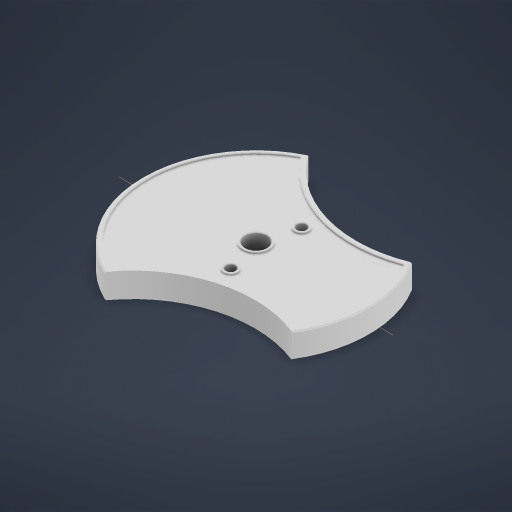
# Autodesk Inventor part: Disk
Saved by Autodesk Inventor 2023.2 (Build 272271000, 271)
## iProperties
Created: 2022-11-28
Part Number: Disk
Material: Generic
Document SubType Name: Modeling
Designer: iusti
Density: 1 g/cm^3
Appearance: Gunmetal - Antique Polished
Author: iusti
Autodesk Inventor part; units mm, degrees
ref_plane "YZ Plane" through (0, 0, 0) normal (1, 0, 0) x (0, 1, 0)
ref_plane "XZ Plane" through (0, 0, 0) normal (0, 1, 0) x (-1, 0, 0)
ref_plane "XY Plane" through (0, 0, 0) normal (0, 0, 1) x (1, 0, 0)
sketch "Sketch1" plane through (0, 0, 0) normal (0, 1, 0) x (-1, 0, 0)
  arc A0 (-38.9896, 24.4092) -> (-38.9896, -24.4092) centre (0, 0) ccw
  arc A1 (-38.9896, 24.4092) -> (20.1302, 41.3615) centre (-20.1215, 70.1721) ccw
  line L0 (0, 0) -> (-20.1215, 70.1721) construction
  line L1 (102.2, 0) -> (-102.2, 0) construction
  circle A2 centre (0, 0) radius 73 construction
  arc A3 (20.1302, -41.3615) -> (-38.9896, -24.4092) centre (-20.1215, -70.1721) ccw
  line L2 (20.1302, 41.3615) -> (20.1302, -41.3615) construction
  line L3 (-38.9896, 24.4092) -> (-38.9896, -24.4092) construction
  arc A4 (-12.6793, 44.218) -> (-38.9896, 24.4092) centre (0, 0) ccw construction
  arc A5 (20.1302, 41.3615) -> (-12.6793, 44.218) centre (0, 0) ccw construction
  arc A6 (20.1302, -41.3615) -> (20.1302, 41.3615) centre (0, 0) ccw
  arc A7 (-38.9896, -24.4092) -> (20.1302, -41.3615) centre (0, 0) ccw construction
  dimension "d3" = 146
  dimension "d0" = 92
  dimension "d1" = 49.5
  dimension "d2" = 74
  constraints: 14 point on circle, 7 centre point, 6 end point, 3 coincident, 3 symmetric about line, 2 vertical, 1 point on line, 4 other
  measures "d0" diameter of A0
  measures "d1" radius of A1
  measures "d2" angle of L1 L0
extrude "Extrusion1" add sketch "Sketch1" along normal mid plane 10
sketch "Sketch6" plane through (0, 5, 0) normal (0, 1, 0) x (1, 0, 0)
  arc A0 (-20.1302, 41.3615) -> (-20.1302, -41.3615) centre (0, 0) ccw projected
  arc A1 (38.9896, -24.4092) -> (-20.1302, -41.3615) centre (20.1215, -70.1721) ccw projected
  arc A2 (38.9896, -24.4092) -> (38.9896, 24.4092) centre (0, 0) ccw projected
  arc A3 (-20.1302, 41.3615) -> (38.9896, 24.4092) centre (20.1215, 70.1721) ccw projected
  line L0 (0, 0) -> (20.1215, -70.1721) construction
  line L1 (0, 0) -> (20.1215, 70.1721) construction
  point P0 (4.1346, -14.4189)
  point P1 (4.1346, 14.4189)
  dimension "d15" = 15
  constraints: 4 end point, 2 point on line, 1 vertical alignment
  measures "d15" distance of point (4.135, -14.419) A0.centre
hole "Hole1" at (4.1346, 5, 14.4189) at (4.1346, 5, -14.4189) direction (0, -1, 0) diameter 4 end through all
sketch "Sketch7" plane through (0, 5, 0) normal (0, 1, 0) x (1, 0, 0)
  circle A0 centre (4.1346, -14.4189) radius 2 projected
  circle A1 centre (4.1346, 14.4189) radius 2 projected
  arc A2 (-20.1302, 41.3615) -> (-20.1302, -41.3615) centre (0, 0) ccw projected
  arc A3 (38.9896, -24.4092) -> (-20.1302, -41.3615) centre (20.1215, -70.1721) ccw projected
  arc A4 (38.9896, -24.4092) -> (38.9896, 24.4092) centre (0, 0) ccw projected
  arc A5 (-20.1302, 41.3615) -> (38.9896, 24.4092) centre (20.1215, 70.1721) ccw projected
  arc A6 (-20.7288, 38.8113) -> (-20.7288, -38.8113) centre (0, 0) ccw
  arc A7 (-20.7288, 38.8113) -> (38.1459, 21.9293) centre (20.1215, 70.1721) ccw
  arc A8 (38.1459, -21.9293) -> (38.1459, 21.9293) centre (0, 0) ccw
  arc A9 (38.1459, -21.9293) -> (-20.7288, -38.8113) centre (20.1215, -70.1721) ccw
  circle A10 centre (4.1346, -14.4189) radius 3
  circle A11 centre (4.1346, 14.4189) radius 3
  circle A12 centre (0, 0) radius 5.5
  dimension "d23" = 2
  dimension "d24" = 6
  dimension "d25" = 6
  dimension "d35" = 11
  constraints: 8 point on circle, 7 centre point, 3 coincident, 3 other
  measures "d23" radial gap between concentric circles of A3 A9
  measures "d24" diameter of A10
  measures "d25" diameter of A11
  measures "d35" diameter of A12
extrude "Extrusion3" cut sketch "Sketch7" against normal blind 0.5 contours A7 A8 A9 A6
hole "Hole2" at (0, 5, 0) direction (0, -1, 0) diameter 9 end through all
chamfer "Chamfer2" distance 0.5 angle 45 2 edges at (-46, 5, 0) (46, 5, 0)
mirror "Mirror2" about plane through (0, 0, 0) normal (0, 1, 0) of "Extrusion3"
chamfer "Chamfer3" distance 0.5 angle 45 2 edges at (46, -5, 0) (-46, -5, 0)
body "Solid1"
